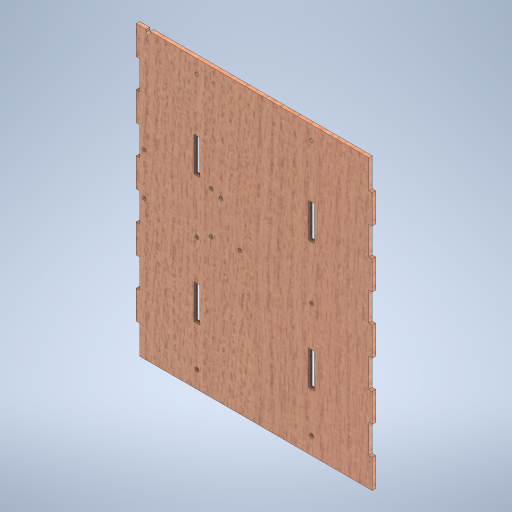
# Autodesk Inventor part: Envolvente_Pared_Trasera
Saved by Autodesk Inventor 2024 (Build 280153000, 153)
## iProperties
Created: 2024-07-16
Part Number: Envolvente_Pared_Trasera
Material: Genérico
Document SubType Name: Modeling
Designer: sergi
Density: 1 g/cm^3
Appearance: Valor por defecto
Author: sergi
Autodesk Inventor part; units mm, degrees
ref_plane "YZ Plane" through (0, 0, 0) normal (1, 0, 0) x (0, 1, 0)
ref_plane "XZ Plane" through (0, 0, 0) normal (0, 1, 0) x (-1, 0, 0)
ref_plane "XY Plane" through (0, 0, 0) normal (0, 0, 1) x (1, 0, 0)
sketch "Boceto1" plane through (0, 0, 0) normal (0, 0, 1) x (1, 0, 0)
  line L0 (206, -30) -> (206, 220) projected
  line L1 (0, 220) -> (206, 220) projected
  line L2 (0, -30) -> (0, 220) projected
  line L3 (206, -30) -> (0, -30) projected
  line L4 (206, -30) -> (206, -5)
  line L5 (206, -5) -> (203, -5)
  line L6 (203, -5) -> (203, 20)
  line L7 (203, 20) -> (206, 20)
  line L8 (206, 20) -> (206, 45)
  line L9 (206, 45) -> (203, 45)
  line L10 (203, 45) -> (203, 70)
  line L11 (203, 70) -> (206, 70)
  line L12 (206, 70) -> (206, 95)
  line L13 (206, 95) -> (203, 95)
  line L14 (203, 95) -> (203, 120)
  line L15 (203, 120) -> (206, 120)
  line L16 (206, 120) -> (206, 145)
  line L17 (206, 145) -> (203, 145)
  line L18 (203, 145) -> (203, 170)
  line L19 (203, 170) -> (206, 170)
  line L20 (203, 220) -> (206, 220)
  line L21 (206, 195) -> (203, 195)
  line L22 (203, 195) -> (203, 220)
  line L23 (206, 170) -> (206, 195)
  line L24 (203, 170) -> (206, 170)
  line L25 (0, 220) -> (0, 195)
  line L26 (0, 195) -> (3, 195)
  line L27 (3, 195) -> (3, 170)
  line L28 (3, 170) -> (0, 170)
  line L29 (0, 170) -> (0, 145)
  line L30 (0, 145) -> (3, 145)
  line L31 (3, 145) -> (3, 120)
  line L32 (3, 120) -> (0, 120)
  line L33 (3, 20) -> (0, 20)
  line L34 (0, 45) -> (3, 45)
  line L35 (3, 45) -> (3, 20)
  line L36 (0, 70) -> (0, 45)
  line L37 (3, 70) -> (0, 70)
  line L38 (3, 95) -> (3, 70)
  line L39 (0, 95) -> (3, 95)
  line L40 (0, 120) -> (0, 95)
  line L41 (3, 20) -> (0, 20)
  line L42 (0, 20) -> (0, -5)
  line L43 (0, -5) -> (3, -5)
  line L44 (3, -5) -> (3, -30)
  line L45 (3, -30) -> (0, -30)
  line L46 (203, 220) -> (206, 220)
  line L47 (203, 220) -> (206, 220)
  line L48 (206, 220) -> (206, 245)
  line L49 (206, 245) -> (203, 245)
  line L50 (203, 245) -> (203, 270)
  line L51 (203, 270) -> (206, 270)
  line L52 (0, 220) -> (3, 220)
  line L53 (0, 220) -> (3, 220)
  line L54 (3, 220) -> (3, 245)
  line L55 (3, 245) -> (0, 245)
  line L56 (0, 245) -> (0, 270)
  line L57 (0, 270) -> (3, 270)
  line L58 (206, 270) -> (0, 270)
  point P0 (0, 0)
  dimension "d78" = 3
  dimension "d88" = 3
  dimension "Lengueta" = 25
  dimension "espesor" = 3
  dimension "d2" = 25
  dimension "d3" = 3
  dimension "d4" = 25
  dimension "d5" = 90
  dimension "d6" = 3
  dimension "d7" = 25
  dimension "d8" = 3
  dimension "d9" = 25
  dimension "d10" = 3
  dimension "d11" = 25
  dimension "d12" = 3
  dimension "d13" = 25
  dimension "d14" = 90
  dimension "d15" = 3
  dimension "d16" = 25
  dimension "d17" = 3
  dimension "d18" = 3
  dimension "d19" = 25
  dimension "d20" = 90
  dimension "d21" = 3
  dimension "d22" = 25
  dimension "d23" = 3
  dimension "d26" = 25
  dimension "d27" = 3
  dimension "d28" = 25
  dimension "d29" = 3
  dimension "d30" = 25
  dimension "d31" = 90
  dimension "d32" = 3
  dimension "d33" = 25
  dimension "d34" = 3
  dimension "d35" = 25
  dimension "d36" = 3
  dimension "d37" = 25
  dimension "d38" = 3
  dimension "d39" = 25
  dimension "d40" = 90
  dimension "d41" = 3
  dimension "d42" = 25
  dimension "d43" = 3
  dimension "d44" = 3
  dimension "d45" = 25
  dimension "d46" = 90
  dimension "d47" = 3
  dimension "d48" = 25
  dimension "d49" = 3
  dimension "d71" = 3
  dimension "d72" = 3
  dimension "d73" = 25
  dimension "d74" = 90
  dimension "d75" = 3
  dimension "d76" = 25
  dimension "d77" = 3
  dimension "d81" = 3
  dimension "d82" = 3
  dimension "d83" = 25
  dimension "d84" = 90
  dimension "d85" = 3
  dimension "d86" = 25
  dimension "d87" = 3
  constraints: 110 end point, 16 perpendicular, 7 point on line, 5 vertical
  measures "Lengueta" distance of L0.start L4.end
  measures "espesor" distance of L4.end L5.end
  measures "d2" distance of L5.end L6.end
  measures "d3" distance of L6.end L7.end
  measures "d4" distance of L7.end L8.end
  measures "d5" angle of L8 L7
  measures "d6" distance of L8.end L9.end
  measures "d7" distance of L9.end L10.end
  measures "d8" distance of L10.end L11.end
  measures "d9" distance of L12.start L13.start
  measures "d10" distance of L13.start L14.start
  measures "d11" distance of L14.start L15.start
  measures "d12" distance of L15.start L16.start
  measures "d13" distance of L16.start L17.start
  measures "d14" angle of L16 L15
  measures "d15" distance of L17.start L17.end
  measures "d16" distance of L17.end L19.start
  measures "d17" distance of L19.start L19.end
  measures "d18" distance of L24.start L24.end
  measures "d19" distance of L24.end L23.end
  measures "d20" angle of L23 L24
  measures "d21" distance of L23.end L21.end
  measures "d22" distance of L21.end L22.end
  measures "d23" distance of L22.end L20.end
  measures "d26" distance of L25.start L25.end
  measures "d27" distance of L25.end L27.start
  measures "d28" distance of L27.start L28.start
  measures "d29" distance of L28.start L28.end
  measures "d30" distance of L28.end L29.end
  measures "d31" angle of L29 L28
  measures "d32" distance of L29.end L30.end
  measures "d33" distance of L30.end L32.start
  measures "d34" distance of L32.start L32.end
  measures "d35" distance of L40.start L39.start
  measures "d36" distance of L39.start L39.end
  measures "d37" distance of L39.end L37.start
  measures "d38" distance of L37.start L37.end
  measures "d39" distance of L37.end L34.start
  measures "d40" angle of L36 L37
  measures "d41" distance of L34.start L34.end
  measures "d42" distance of L34.end L35.end
  measures "d43" distance of L35.end L33.end
  measures "d44" distance of L41.start L41.end
  measures "d45" distance of L41.end L42.end
  measures "d46" angle of L42 L41
  measures "d47" distance of L42.end L43.end
  measures "d48" distance of L43.end L44.end
  measures "d49" distance of L44.end L45.end
  measures "d71" distance of L46.start L46.end
  measures "d72" distance of L47.start L47.end
  measures "d73" distance of L47.end L49.start
  measures "d74" angle of L48 L47
  measures "d75" distance of L49.start L49.end
  measures "d76" distance of L49.end L50.end
  measures "d77" distance of L50.end L51.end
  measures "d81" distance of L52.start L52.end
  measures "d82" distance of L53.start L53.end
  measures "d83" distance of L53.end L55.start
  measures "d84" angle of L54 L53
  measures "d85" distance of L55.start L55.end
  measures "d86" distance of L55.end L56.end
  measures "d87" distance of L56.end L57.end
extrude "Extrusión1" add sketch "Boceto1" against normal blind 3 contours L3 L44 L43 L2 L33 L35 L34 L37 L38 L39 L32 L31 L30 L28 L27 L26 L1 L22 L21 L0 L19 L18 L17 L15 L14 L13 L11 L10 L9 L7 L6 L5
sketch "Boceto2" plane through (0, 0, 0) normal (0, 0, 1) x (1, 0, 0)
  circle A0 centre (53, -15) radius 1.75
  circle A1 centre (153, -15) radius 1.75
  point P0 (0, 0)
  constraints: 2 centre point, 4 other
extrude "Extrusión2" cut sketch "Boceto2" against normal blind 3
sketch "Boceto3" plane through (0, 0, 0) normal (0, 0, 1) x (1, 0, 0)
  circle A0 centre (53, 208) radius 2.1
  circle A1 centre (53, 208) radius 1.5
  circle A2 centre (153, 208) radius 2.1
  point P0 (0, 0)
  dimension "d56" = 3
  constraints: 3 centre point, 1 coincident, 4 other
  measures "d56" diameter of A1
hole "Agujero1" at (53, 208, 0) at (153, 208, 0) direction (0, 0, -1) diameter 3 depth 4
sketch "Boceto4" plane through (0, 0, 0) normal (0, 0, 1) x (1, 0, 0)
  circle A0 centre (53, 85) radius 2.1 projected
  circle A1 centre (153, 85) radius 2.1 projected
  point P0 (0, 0)
hole "Agujero2" at (153, 85, 0) at (53, 85, 0) direction (0, 0, -1) diameter 3 depth 4
sketch "Boceto5" plane through (0, 0, -3) normal (0, 0, -1) x (-1, 0, 0)
  point P0 (0, 0)
sketch "Boceto6" plane through (0, 0, 0) normal (0, 0, 1) x (1, 0, 0)
  circle A0 centre (53, 85) radius 1.5 projected
  circle A1 centre (153, 85) radius 1.5 projected
  circle A2 centre (153, 208) radius 1.5 projected
  circle A3 centre (53, 208) radius 1.5 projected
  circle A4 centre (53, -15) radius 1.75 projected
  circle A5 centre (153, -15) radius 1.75 projected
  line L0 (203, 20) -> (206, 20) projected
  line L1 (206, 20) -> (206, 45) projected
  line L2 (206, 45) -> (203, 45) projected
  line L3 (203, 45) -> (203, 70) projected
  line L4 (203, 70) -> (206, 70) projected
  line L5 (206, 70) -> (206, 95) projected
  line L6 (206, 95) -> (203, 95) projected
  line L7 (203, 95) -> (203, 120) projected
  line L8 (203, 120) -> (206, 120) projected
  line L9 (206, 120) -> (206, 145) projected
  line L10 (206, 145) -> (203, 145) projected
  line L11 (203, 145) -> (203, 170) projected
  line L12 (203, 170) -> (206, 170) projected
  line L13 (206, 170) -> (206, 195) projected
  line L14 (206, 195) -> (203, 195) projected
  line L15 (203, 195) -> (203, 220) projected
  line L16 (203, 220) -> (0, 220) projected
  line L17 (0, 220) -> (0, 195) projected
  line L18 (0, 195) -> (3, 195) projected
  line L19 (3, 195) -> (3, 170) projected
  line L20 (3, 170) -> (0, 170) projected
  line L21 (0, 170) -> (0, 145) projected
  line L22 (0, 145) -> (3, 145) projected
  line L23 (3, 145) -> (3, 120) projected
  line L24 (3, 120) -> (0, 120) projected
  line L25 (0, 120) -> (0, 95) projected
  line L26 (0, 95) -> (3, 95) projected
  line L27 (3, 95) -> (3, 70) projected
  line L28 (3, 70) -> (0, 70) projected
  line L29 (0, 70) -> (0, 45) projected
  line L30 (0, 45) -> (3, 45) projected
  line L31 (3, 45) -> (3, 20) projected
  line L32 (3, 20) -> (0, 20) projected
  line L33 (0, 20) -> (0, -5) projected
  line L34 (0, -5) -> (3, -5) projected
  line L35 (3, -5) -> (3, -30) projected
  line L36 (3, -30) -> (206, -30) projected
  line L37 (206, -30) -> (206, -5) projected
  line L38 (206, -5) -> (203, -5) projected
  line L39 (203, -5) -> (203, 20) projected
  line L40 (153, 85) -> (153, 208)
  line L41 (150.5, 161.5) -> (155.5, 161.5)
  line L42 (155.5, 161.5) -> (155.5, 131.5)
  line L43 (155.5, 131.5) -> (150.5, 131.5)
  line L44 (150.5, 131.5) -> (150.5, 161.5)
  line L45 (150.5, 161.5) -> (155.5, 131.5) construction
  line L46 (155.5, 161.5) -> (150.5, 131.5) construction
  line L47 (53, 85) -> (53, 208)
  line L48 (50.5, 161.5) -> (55.5, 161.5)
  line L49 (55.5, 161.5) -> (55.5, 131.5)
  line L50 (55.5, 131.5) -> (50.5, 131.5)
  line L51 (50.5, 131.5) -> (50.5, 161.5)
  line L52 (50.5, 161.5) -> (55.5, 131.5) construction
  line L53 (55.5, 161.5) -> (50.5, 131.5) construction
  line L54 (53, -15) -> (53, 85)
  line L55 (50.5, 50) -> (55.5, 50)
  line L56 (55.5, 50) -> (55.5, 20)
  line L57 (55.5, 20) -> (50.5, 20)
  line L58 (50.5, 20) -> (50.5, 50)
  line L59 (50.5, 50) -> (55.5, 20) construction
  line L60 (55.5, 50) -> (50.5, 20) construction
  line L61 (150.5, 50) -> (155.5, 50)
  line L62 (155.5, 50) -> (155.5, 20)
  line L63 (155.5, 20) -> (150.5, 20)
  line L64 (150.5, 20) -> (150.5, 50)
  line L65 (150.5, 50) -> (155.5, 20) construction
  line L66 (155.5, 50) -> (150.5, 20) construction
  point P0 (0, 0)
  point P1 (153, 146.5)
  point P2 (53, 146.5)
  point P3 (53, 35)
  point P4 (153, 35)
  dimension "d93" = 5
  dimension "d94" = 30
  dimension "d95" = 5
  dimension "d96" = 30
  dimension "d99" = 5
  dimension "d100" = 30
  dimension "d101" = 5
  dimension "d102" = 30
  constraints: 54 end point, 11 midpoint, 8 parallel, 4 horizontal, 4 perpendicular, 3 vertical
  measures "d93" distance of L42.end L43.end
  measures "d94" distance of L41.end L42.end
  measures "d95" distance of L50.start L50.end
  measures "d96" distance of L48.end L50.start
  measures "d99" distance of L56.end L57.end
  measures "d100" distance of L55.end L56.end
  measures "d101" distance of L62.end L63.end
  measures "d102" distance of L62.start L62.end
extrude "Extrusión3" cut sketch "Boceto6" against normal blind 3 contours L55 L56 L57 L54 | L54 L57 L58 L55 | L50 L51 L48 L47 | L47 L48 L49 L50 | L43 L44 L41 L40 | L40 L41 L42 L43 | L61 L62 L63 L64
sketch "Boceto7" plane through (0, 0, 0) normal (0, 0, 1) x (1, 0, 0)
  line L0 (3, 95.5) -> (60.5, 95.5) projected
  line L1 (60.5, 95.5) -> (60.5, 98.5) projected
  line L2 (60.5, 98.5) -> (3, 98.5) projected
  line L3 (3, 98.5) -> (3, 121) projected
  line L4 (3, 121) -> (60.5, 121) projected
  line L5 (60.5, 121) -> (60.5, 124) projected
  line L6 (60.5, 124) -> (3, 124) projected
  line L7 (3, 124) -> (3, 128) projected
  arc A0 (10.873, 129) -> (3, 128) centre (7, 128) ccw projected
  arc A1 (10.873, 129) -> (14.746, 126) centre (14.746, 130) ccw projected
  line L8 (14.746, 126) -> (57.754, 126) projected
  arc A2 (57.754, 126) -> (61.627, 129) centre (57.754, 130) ccw projected
  arc A3 (69.5, 128) -> (61.627, 129) centre (65.5, 128) ccw projected
  line L9 (69.5, 128) -> (69.5, 91.5) projected
  arc A4 (61.627, 90.5) -> (69.5, 91.5) centre (65.5, 91.5) ccw projected
  arc A5 (61.627, 90.5) -> (57.754, 93.5) centre (57.754, 89.5) ccw projected
  line L10 (57.754, 93.5) -> (14.746, 93.5) projected
  arc A6 (14.746, 93.5) -> (10.873, 90.5) centre (14.746, 89.5) ccw projected
  arc A7 (3, 91.5) -> (10.873, 90.5) centre (7, 91.5) ccw projected
  line L11 (3, 91.5) -> (3, 95.5) projected
  line L12 (66.1403, 93.5) -> (64.8597, 93.5) projected
  arc A8 (64.8597, 93.5) -> (66.1403, 93.5) centre (65.5, 91.5) ccw projected
  arc A9 (66.1403, 126) -> (64.8597, 126) centre (65.5, 128) ccw projected
  line L13 (64.8597, 126) -> (66.1403, 126) projected
  line L14 (6.3597, 126) -> (7.6403, 126) projected
  arc A10 (7.6403, 126) -> (6.3597, 126) centre (7, 128) ccw projected
  arc A11 (6.3597, 93.5) -> (7.6403, 93.5) centre (7, 91.5) ccw projected
  line L15 (7.6403, 93.5) -> (6.3597, 93.5) projected
  circle A12 centre (74.05, 124.85) radius 1.55 projected
  circle A13 centre (90.35, 93.75) radius 1.55 projected
  line L16 (92.9, 87.6) -> (71.5, 87.6) projected
  line L17 (71.5, 87.6) -> (71.5, 131) projected
  line L18 (71.5, 131) -> (92.9, 131) projected
  line L19 (92.9, 131) -> (92.9, 87.6) projected
  point P0 (0, 0)
hole "Agujero3" at (65.5, 128, 0) at (7, 128, 0) at (7, 91.5, 0) at (65.5, 91.5, 0) at (90.35, 93.75, 0) at (74.05, 124.85, 0) direction (0, 0, -1) diameter 3.1 end through all
sketch "Boceto8" plane through (0, 0, 0) normal (0, 0, 1) x (1, 0, 0)
  line L0 (0, 220) -> (203, 220) projected
  line L1 (0, 220) -> (3, 220)
  line L2 (3, 220) -> (18, 220)
  line L3 (18, 220) -> (18, 205)
  line L4 (18, 205) -> (3, 205)
  line L5 (3, 205) -> (3, 220)
  line L6 (16.3, 206.7) -> (16.3, 218.3)
  line L7 (16.3, 218.3) -> (4.7, 218.3)
  line L8 (4.7, 218.3) -> (4.7, 206.7)
  line L9 (4.7, 206.7) -> (16.3, 206.7)
  circle A0 centre (10.5, 218.3) radius 1.7
  line L10 (12.2, 218.3) -> (12.2, 220)
  line L11 (8.8, 218.3) -> (8.8, 220)
  point P0 (0, 0)
  dimension "d115" = 3
  dimension "d116" = 15
  dimension "d117" = 15
  dimension "d118" = 1.7
  dimension "d119" = 3.4
  constraints: 22 end point, 5 point on line, 4 parallel, 4 perpendicular, 2 point on circle, 2 tangent, 1 centre point, 1 horizontal, 1 midpoint, 3 other
  measures "d115" distance of L0.start L1.end
  measures "d116" distance of L3.end L4.end
  measures "d117" distance of L2.end L3.end
  measures "d118" distance between parallel lines of L3 L6
  measures "d119" diameter of A0
extrude "Extrusión4" cut sketch "Boceto8" against normal blind 10 contours L0 A0 L11 | L0 L10 A0 | A0 L7 | L7 A0
equation "\"d2\" = Lengueta"
equation "\"d3\" = espesor"
equation "\"d4\" = Lengueta"
equation "\"d6\" = espesor"
equation "\"d7\" = Lengueta"
equation "\"d8\" = espesor"
equation "\"d11\" = d9"
equation "\"d12\" = d10"
equation "\"d13\" = d9"
equation "\"d16\" = d9"
equation "\"d18\" = d24"
equation "\"d19\" = d25"
equation "\"d22\" = d25"
equation "\"d28\" = d26"
equation "\"d29\" = d27"
equation "\"d30\" = d26"
equation "\"d33\" = d26"
equation "\"d37\" = d35"
equation "\"d38\" = d36"
equation "\"d39\" = d35"
equation "\"d42\" = d35"
equation "\"d44\" = d50"
equation "\"d45\" = d51"
equation "\"d48\" = d51"
equation "\"d71\" = d78"
equation "\"d72\" = d79"
equation "\"d73\" = d80"
equation "\"d76\" = d80"
equation "\"d81\" = d88"
equation "\"d82\" = d89"
equation "\"d83\" = d90"
equation "\"d86\" = d90"
equation "\"d52\" = espesor"
equation "\"d54\" = espesor"
equation "\"d24\" = 3"
equation "\"d25\" = 25"
equation "\"d50\" = 3"
equation "\"d51\" = 25"
equation "\"d79\" = 3"
equation "\"d80\" = 25"
equation "\"d89\" = 3"
equation "\"d90\" = 25"
